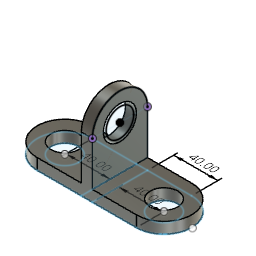
ex53 (Autodesk Fusion 360 design; units mm, degrees)
Autodesk Fusion 360 part; units mm, degrees
sketch "Sketch1" plane through (0, 0, 0) normal (0, 0, 1) x (1, 0, 0)
  line L0 (-5, 0) -> (-5, -50)
  line L1 (5, 0) -> (5, -50)
  line L2 (5, 0) -> (45, 0)
  line L3 (-5, 0) -> (-45, 0)
  line L4 (5, -50) -> (45, -50)
  line L5 (-5, -50) -> (-45, -50)
  line L6 (70, -25) -> (70.7973, -25) construction
  circle A0 centre (-45, -25) radius 12.5
  circle A1 centre (45, -25) radius 12.5
  arc A2 (-45, 0) -> (-45, -50) centre (-45, -25) ccw
  arc A3 (45, -50) -> (45, 0) centre (45, -25) ccw
  line L7 (-5, 0) -> (5, 0)
  line L8 (-5, -50) -> (5, -50)
  dimension "d4" = 40
  dimension "d5" = 40
  dimension "d6" = 40
  dimension "d7" = 40
  dimension "d8" = 25
  dimension "d9" = 50
  dimension "d10" = 25
  dimension "d11" = 50
  constraint perpendicular L1 L2
  constraint perpendicular L0 L3
  constraint perpendicular L1 L4
  constraint perpendicular L0 L5
  constraint concentric A0 A2
  constraint concentric A1 A3
  constraint coincident A3 L6.start
  constraint perpendicular L1 L7
  constraint perpendicular L1 L8
  measures "d4" distance of L1.start L2.end
  measures "d5" distance of L0.start L3.end
  measures "d6" distance of L1.end L4.end
  measures "d7" distance of L0.end L5.end
  measures "d8" diameter of A0
  measures "d9" diameter of A2
  measures "d10" diameter of A1
  measures "d11" diameter of A3
extrude "Extrude1" add sketch "Sketch1" along normal blind 10 contours L0 L3 L5 A2 | L1 L2 L4 A3 makes body 1 at (-14.1667, -25, 0) makes body 2 at (14.1667, -25, 0)
extrude "Extrude2" add sketch "Sketch1" along normal blind 50 contours L0 L1 L7 L8 bodies 1 2
sketch "Sketch2" plane through (5, 0, 0) normal (1, 0, 0) x (0, 1, 0)
  line L0 (-50, 10) -> (0, 10)
  line L1 (0, 10) -> (0, 50)
  line L2 (0, 50) -> (-50, 50)
  line L3 (-50, 50) -> (-50, 10)
  arc A0 (0, 50) -> (-50, 50) centre (-25, 50) ccw
  circle A1 centre (-25, 50) radius 12.5
  dimension "d16" = 50
  dimension "d17" = 25
  constraint midpoint L2 A0.centre
  constraint concentric A0 A1
  measures "d16" diameter of A0
  measures "d17" diameter of A1
extrude "Extrude3" add sketch "Sketch2" against normal blind 10 contours L2 A0 A1 bodies 1
hole "Hole1" at (5, -25, 50) direction (-1, 0, 0) diameter 30 depth 30 tip angle 118 bodies 1
